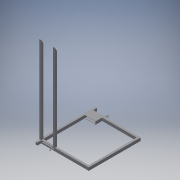
# Autodesk Inventor part: Zijplaat 1
Saved by Autodesk Inventor 2018.3 (Build 223284000, 284)
## iProperties
Created: 2020-11-16
Part Number: Zijplaat 1
Material: Generic
Document SubType Name: Modeling
Designer: daanv
Density: 1 g/cm^3
Appearance: Default
Author: daanv
Autodesk Inventor part; units mm, degrees
ref_plane "YZ Plane" through (0, 0, 0) normal (1, 0, 0) x (0, 1, 0)
ref_plane "XZ Plane" through (0, 0, 0) normal (0, 1, 0) x (-1, 0, 0)
ref_plane "XY Plane" through (0, 0, 0) normal (0, 0, 1) x (1, 0, 0)
sketch "Sketch1" plane through (0, 0, 0) normal (0, 0, 1) x (1, 0, 0)
  line L0 (0, 0) -> (50, 0)
  line L1 (50, 0) -> (50, 52.5)
  line L2 (50, 52.5) -> (0, 52.5)
  line L3 (0, 52.5) -> (0, 0)
  dimension "d0" = 50
  dimension "d1" = 52.5
  constraints: 8 end point, 2 parallel, 1 horizontal, 1 perpendicular
  measures "d0" distance of L2.end L1.end
  measures "d1" distance of L1.end L0.end
extrude "Extrusion1" add sketch "Sketch1" along normal blind 3
sketch "Sketch2" plane through (0, 0, 3) normal (0, 0, 1) x (1, 0, 0)
  line L0 (2, 50.5) -> (48, 50.5)
  line L1 (48, 50.5) -> (48, 2)
  line L2 (48, 2) -> (2, 2)
  line L3 (2, 2) -> (2, 50.5)
  dimension "d4" = 46
  dimension "d5" = 48.5
  constraints: 8 end point, 2 parallel, 1 horizontal, 1 perpendicular
  measures "d4" distance of L1.end L2.end
  measures "d5" distance of L0.end L1.end
extrude "Extrusion2" cut sketch "Sketch2" against normal blind 10
sketch "Sketch3" plane through (0, 0, 3) normal (0, 0, 1) x (1, 0, 0)
  line L0 (48, 2) -> (2, 2) projected
  line L1 (0, 52.5) -> (0, 0) projected
  line L2 (2, 2) -> (0, 2)
  line L3 (0, 2) -> (0, 0)
  line L4 (0, 0) -> (2, 0)
  line L5 (2, 0) -> (2, 2)
  line L6 (0, 0) -> (50, 0) projected
  line L7 (13.7, 2) -> (15.7, 2)
  line L8 (15.7, 2) -> (15.7, 0)
  line L9 (15.7, 0) -> (13.7, 0)
  line L10 (13.7, 0) -> (13.7, 2)
  line L11 (0, 2) -> (2, 2)
  line L12 (2, 2) -> (2, 0)
  line L13 (2, 0) -> (0, 0)
  line L14 (0, 0) -> (0, 2)
  line L15 (13.7, 2) -> (15.7, 2)
  line L16 (15.7, 2) -> (15.7, 0)
  line L17 (15.7, 0) -> (13.7, 0)
  line L18 (13.7, 0) -> (13.7, 2)
  dimension "d8" = 2
  dimension "d9" = 11.7
  constraints: 32 end point, 9 parallel, 4 horizontal, 4 perpendicular, 2 point on line
  measures "d8" distance of L8.end L9.end
  measures "d9" distance between parallel lines of L5 L10
extrude "Extrusion3" add sketch "Sketch3" along normal blind 87.5 contours L8 L6 L10 L0 | L5 L4 L1 L2
chamfer "Chamfer1" distance 2 angle 60 1 edges at (1, 2, 90.5) measured on face at (1.3333, 0.6667, 90.5)
chamfer "Chamfer2" distance 2 angle 60 1 edges at (14.7, 2, 90.5) measured on face at (14.3667, 0.6667, 90.5)
sketch "Sketch4" plane through (0, 0, 0) normal (0, -1, 0) x (1, 0, 0)
  line L0 (0, 0) -> (50, 0) projected
  line L1 (0, 0) -> (0, 90.5) projected
  line L2 (12.85, 1.5) -> (2.85, 1.5)
  line L3 (2.85, 1.5) -> (2.85, 2.5)
  line L4 (2.85, 2.5) -> (12.85, 2.5)
  line L5 (12.85, 2.5) -> (12.85, 1.5)
  dimension "d18" = 10
  dimension "d19" = 1
  dimension "d20" = 1.5
  dimension "d21" = 2.85
  constraints: 8 end point, 2 parallel, 1 horizontal, 1 perpendicular
  measures "d18" distance of L3.end L4.end
  measures "d19" distance of L2.end L3.end
  measures "d20" distance between parallel lines of L0 L2
  measures "d21" distance between parallel lines of L1 L3
extrude "Extrusion4" cut sketch "Sketch4" against normal blind 10
sketch "Sketch5" plane through (0, 0, 0) normal (0, -1, 0) x (1, 0, 0)
  line L0 (12.85, 2.5) -> (12.85, 1.5) projected
  line L1 (2.85, 1.5) -> (2.85, 2.5) projected
  line L2 (0, 0) -> (50, 0) projected
  line L3 (14.1, 2.5) -> (14.966, 2)
  line L4 (14.966, 2) -> (14.1, 1.5)
  line L5 (14.1, 1.5) -> (14.1, 2.5)
  line L6 (2, 3) -> (48, 3) projected
  line L7 (2, 2.8) -> (0.2, 2.8)
  line L8 (0.2, 2.8) -> (0.2, 0.2)
  line L9 (0.2, 0.2) -> (2, 0.2)
  line L10 (2, 0.2) -> (2, 2.8)
  line L11 (2, 3) -> (13.7, 3) projected
  dimension "d24" = 1
  dimension "d25" = 1.8
  dimension "d26" = 0.85
  dimension "d27" = 1.25
  dimension "d28" = 1.8
  dimension "d29" = 2.6
  dimension "d30" = 2.6
  dimension "d31" = 1
  dimension "d32" = 1
  dimension "d33" = 0.5
  dimension "d103" = 0.2
  dimension "d104" = 0.2
  constraints: 14 end point, 4 perpendicular, 1 horizontal
  measures "d24" distance of L3.start L3.end
  measures "d25" distance of L7.start L7.end
  measures "d26" distance between parallel lines of L10 L1
  measures "d27" distance between parallel lines of L0 L5
  measures "d28" distance of L8.end L9.end
  measures "d29" distance of L7.end L8.end
  measures "d30" distance of L9.end L7.start
  measures "d31" distance of L3.end L4.end
  measures "d32" distance of L4.end L3.start
  measures "d33" distance from line of L6 L3.start
  measures "d103" distance between parallel lines of L11 L7
  measures "d104" distance between parallel lines of L2 L9
extrude "Extrusion5" add sketch "Sketch5" along normal blind 4
sketch "Sketch6" plane through (0, 52.5, 0) normal (0, 1, 0) x (1, 0, 0)
  line L0 (0, 0) -> (0, -3) projected
  line L1 (50, -3) -> (0, -3) projected
  line L2 (12.66, -1.75) -> (12.66, -2.77)
  line L3 (12.66, -2.77) -> (2, -2.77)
  line L4 (2, -2.77) -> (2, -0.23)
  line L5 (2, -0.23) -> (12.66, -0.23)
  line L6 (12.66, -0.23) -> (12.66, -2.77)
  line L7 (50, 0) -> (0, 0) projected
  point P0 (2.85, -1.5)
  dimension "d1" = 52.5
  dimension "d51" = 10.66
  dimension "d52" = 2.54
  dimension "d54" = 0.23
  dimension "d55" = 2
  dimension "d57" = 0.23
  constraints: 10 end point, 2 parallel, 1 horizontal, 1 perpendicular
  measures "d51" distance of L4.end L5.end
  measures "d52" distance of L3.end L4.end
  measures "d54" distance between parallel lines of L1 L3
  measures "d55" distance between parallel lines of L0 L4
  measures "d57" distance between parallel lines of L7 L5
extrude "Extrusion6" cut sketch "Sketch6" against normal blind 4
sketch "Sketch7" plane through (2, 50.5, 3) normal (0, -1, 0) x (1, 0, 0)
  line L0 (10.66, -2.77) -> (0, -2.77) projected
  line L1 (46, -3) -> (0, -3) projected
  line L2 (11, -3) -> (0, -3)
  line L3 (0, -3) -> (0, -2.77)
  line L4 (0, 0) -> (11, 0)
  line L5 (0, -0.23) -> (0, 0)
  line L6 (11, 0) -> (11, -3)
  line L7 (10.66, -2.77) -> (0, -2.77)
  line L8 (0, -0.23) -> (10.66, -0.23)
  line L9 (48, 0) -> (-2, 0) projected
  line L10 (10.66, -2.77) -> (10.66, -0.23)
  line L11 (11, -3) -> (11, 0)
  line L12 (10.66, -2.77) -> (10.66, -0.23) projected
  line L13 (10.66, -2.77) -> (10.66, -0.23)
  point P0 (-2, -3)
  constraints: 20 end point, 4 perpendicular, 2 collinear, 2 horizontal, 1 parallel, 1 point on line
extrude "Extrusion7" add sketch "Sketch7" along normal blind 6.5
sketch "Sketch8" plane through (0, 52.5, 0) normal (0, 1, 0) x (1, 0, 0)
  line L0 (50, 0) -> (0, 0) projected
  line L1 (50, 0) -> (50, -3) projected
  line L2 (12.8966, -0.5) -> (14.6286, -1.5)
  line L3 (12.8966, -0.5) -> (14.8966, -0.5) construction
  line L4 (14.6286, -1.5) -> (12.8966, -2.5)
  line L5 (12.66, -2.77) -> (12.66, -0.23) projected
  line L6 (12.8966, -2.5) -> (12.8966, -0.5)
  line L7 (13.0189, -2.1236) -> (13.0189, -0.9087)
  line L8 (13.0189, -0.9087) -> (13.0189, -0.7479)
  line L9 (13.0189, -0.7479) -> (14.3309, -1.5054)
  line L10 (13.0189, -2.1236) -> (13.0189, -2.2521)
  line L11 (13.0189, -2.2521) -> (14.3309, -1.5054)
  dimension "d60" = 2
  dimension "d61" = 30
  dimension "d62" = 2
  dimension "d63" = 60
  dimension "d64" = 0.5
  dimension "d65" = 35.3714
  dimension "d98" = 1.312
  dimension "d99" = 0.1535
  dimension "d100" = 0.1535
  constraints: 18 end point, 2 vertical, 1 equal length, 1 horizontal, 1 point on line
  measures "d60" distance of L2.start L2.end
  measures "d61" angle of L2 L3
  measures "d62" distance of L2.end L4.end
  measures "d63" angle of L2 L4
  measures "d64" distance from line of L0 L2.start
  measures "d65" distance from line of L1 L2.end
  measures "d98" horizontal distance of L10.end L9.end
  measures "d99" distance from line of L4 L10.end
  measures "d100" distance between parallel lines of L2 L9
sketch "Sketch9" plane through (0, 52.5, 0) normal (0, 1, 0) x (1, 0, 0)
  line L0 (50, 0) -> (0, 0) projected
  line L1 (0, 0) -> (0, -3) projected
  line L2 (50, -3) -> (0, -3) projected
  line L3 (2, -2.77) -> (2, -0.23) projected
  line L4 (2, -3) -> (0, -3)
  line L5 (0, -3) -> (0, 0)
  line L6 (0, 0) -> (2, 0)
  line L7 (2, 0) -> (2, -3)
  line L8 (1.75, -2.5) -> (0.25, -2.5)
  line L9 (0.25, -2.5) -> (0.25, -0.5)
  line L10 (0.25, -0.5) -> (1.75, -0.5)
  line L11 (1.75, -0.5) -> (1.75, -2.5)
  dimension "d74" = 2
  dimension "d75" = 3
  dimension "d76" = 0
  dimension "d77" = 0
  dimension "d78" = 0
  dimension "d79" = 0
  dimension "d81" = 1.5
  dimension "d82" = 2
  dimension "d94" = 0.5
  dimension "d95" = 0.25
  constraints: 16 end point, 4 parallel, 2 horizontal, 2 perpendicular
  measures "d74" distance of L5.end L6.end
  measures "d75" distance of L4.end L5.end
  measures "d76" distance between parallel lines of L3 L7
  measures "d77" distance between parallel lines of L2 L4
  measures "d78" distance between parallel lines of L0 L6
  measures "d79" distance between parallel lines of L1 L5
  measures "d81" distance of L9.end L10.end
  measures "d82" distance of L8.end L9.end
  measures "d94" distance between parallel lines of L2 L8
  measures "d95" distance between parallel lines of L3 L11
extrude "Extrusion10" add sketch "Sketch9" along normal blind 4
extrude "Extrusion11" add sketch "Sketch8" along normal blind 4
body "Solid1"
